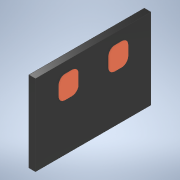
# Autodesk Inventor part: pantalla
Saved by Autodesk Inventor 2021 (Build 250183000, 183)
## iProperties
Created: 2024-10-06
Part Number: pantalla
Material: Generic
Document SubType Name: Modeling
Designer: hojan
Density: 1 g/cm^3
Appearance: Default
Author: hojan
Autodesk Inventor part; units mm, degrees
ref_plane "YZ Plane" through (0, 0, 0) normal (1, 0, 0) x (0, 1, 0)
ref_plane "XZ Plane" through (0, 0, 0) normal (0, 1, 0) x (-1, 0, 0)
ref_plane "XY Plane" through (0, 0, 0) normal (0, 0, 1) x (1, 0, 0)
sketch "Boceto1" plane through (0, 0, 0) normal (1, 0, 0) x (0, 1, 0)
  line L0 (-18.15, 26) -> (18.15, 26)
  line L1 (18.15, 26) -> (18.15, -26)
  line L2 (18.15, -26) -> (-18.15, -26)
  line L3 (-18.15, -26) -> (-18.15, 26)
  line L4 (-18.15, 26) -> (18.15, -26) construction
  line L5 (18.15, 26) -> (-18.15, -26) construction
  point P0 (0, 0)
  dimension "d0" = 36.3
  dimension "d1" = 52
  constraints: 12 end point, 2 midpoint, 2 parallel, 1 horizontal, 1 perpendicular
  measures "d0" distance of L1.end L2.end
  measures "d1" distance of L0.end L1.end
extrude "Extrusión1" add sketch "Boceto1" along normal blind 3
sketch "Boceto2" plane through (3, 0, 0) normal (1, 0, 0) x (0, 0, -1)
  line L0 (-15.7403, 3.1561) -> (-6.6575, 3.1561)
  line L1 (-6.6575, 3.1561) -> (-6.6575, 13.5365)
  line L2 (-6.6575, 13.5365) -> (-15.7403, 13.5365)
  line L3 (-15.7403, 13.5365) -> (-15.7403, 3.1561)
  line L4 (-15.7403, 3.1561) -> (-6.6575, 13.5365) construction
  line L5 (-6.6575, 3.1561) -> (-15.7403, 13.5365) construction
  point P0 (0, 0)
  point P1 (-11.1989, 8.3463)
  constraints: 12 end point, 2 midpoint, 2 parallel, 1 horizontal, 1 perpendicular
extrude "Extrusión2" add sketch "Boceto2" along normal blind 0.1
fillet "Empalme1" radius 3 4 edges at (3.05, 13.5365, 15.7403) (3.05, 13.5365, 6.6575) (3.05, 3.1561, 15.7403) (3.05, 3.1561, 6.6575)
mirror "Simetría1" about plane through (0, 0, 0) normal (0, 0, 1) of "Extrusión2", "Empalme1"
